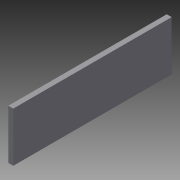
# Autodesk Inventor part: Dish_Front_Base
Saved by Autodesk Inventor 2014 (Build 180170000, 170)
## iProperties
Created: 2015-01-07
Part Number: Dish_Front_Base
Material: Generic
Document SubType Name: Modeling
Designer: Owner
Density: 1 g/cm^3
Appearance: Default
Author: Owner
Autodesk Inventor part; units mm, degrees
ref_plane "YZ Plane" through (0, 0, 0) normal (1, 0, 0) x (0, 1, 0)
ref_plane "XZ Plane" through (0, 0, 0) normal (0, 1, 0) x (-1, 0, 0)
ref_plane "XY Plane" through (0, 0, 0) normal (0, 0, 1) x (1, 0, 0)
sketch "Sketch1" plane through (0, 0, 0) normal (0, 1, 0) x (-1, 0, 0)
  line L0 (39.1686, 27.4724) -> (39.1686, -175.7276)
  line L1 (45.5186, 27.4724) -> (45.5186, -175.7276)
  line L2 (39.1686, -134.4526) -> (39.1686, -137.6276)
  line L3 (39.1686, -175.7276) -> (45.5186, -175.7276)
  line L4 (39.1686, 27.4724) -> (45.5186, 27.4724)
  line L5 (39.1686, -118.5776) -> (39.1686, -121.7526)
  line L6 (39.1686, -12.4056) -> (39.1686, -9.2306)
  point P0 (0, 0)
  dimension "d0" = 6.35
  dimension "d5" = 203.2
  constraints: 14 end point, 3 point on line, 2 perpendicular, 2 vertical
  measures "d0" distance between parallel lines of L1 L0
  measures "d5" distance of L0.start L0.end
extrude "Extrusion1" add sketch "Sketch1" along normal blind 63.5
body "Solid1"
